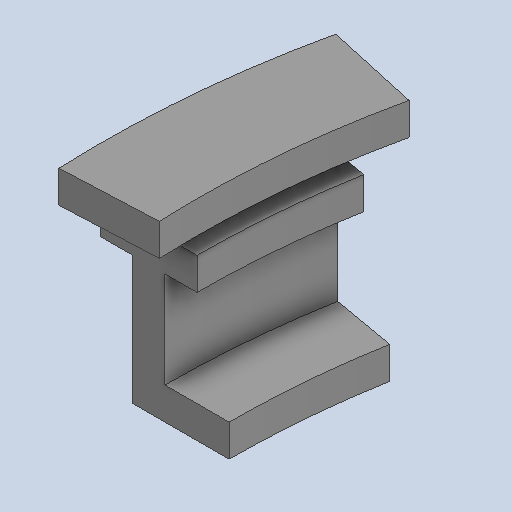
# Autodesk Inventor part: Moving Caoursel base Clip
Saved by Autodesk Inventor 2023 (Build 270158000, 158)
## iProperties
Created: 2023-02-14
Part Number: Moving Caoursel base Clip
Material: PLA Plastic
Document SubType Name: Modeling
Designer: cheng
Density: 1.25002 g/cm^3
Appearance: Generic
Author: cheng
Autodesk Inventor part; units mm, degrees
ref_plane "YZ Plane" through (0, 0, 0) normal (1, 0, 0) x (0, 1, 0)
ref_plane "XZ Plane" through (0, 0, 0) normal (0, 1, 0) x (-1, 0, 0)
ref_plane "XY Plane" through (0, 0, 0) normal (0, 0, 1) x (1, 0, 0)
sketch "Sketch1" plane through (0, 0, 0) normal (0, 1, 0) x (-1, 0, 0)
  circle A0 centre (0, 0) radius 285
  circle A1 centre (0, 0) radius 295
  circle A2 centre (0, 0) radius 275
  circle A3 centre (0, 0) radius 305
  line L0 (0, 0) -> (300.3664, -52.9627)
  line L1 (0, 0) -> (305, 0)
  point P0 (275, 0)
  point P1 (270.8221, -47.7532)
  dimension "d1" = 590
  dimension "d5" = 10
  dimension "d6" = 10
  dimension "d7" = 10
  dimension "d8" = 10
  constraints: 4 centre point, 4 coincident, 4 end point, 2 point on circle, 1 horizontal
  measures "d1" diameter of A1
  measures "d5" radial gap between concentric circles of A2 A0
  measures "d6" radial gap between concentric circles of A1 A0
  measures "d7" radial gap between concentric circles of A1 A3
  measures "d8" angle of L1 L0
extrude "Extrusion1" add sketch "Sketch1" along normal blind 10 contours L1 A1 L0 A0 | A0 L0 A2 L1 | L1 A3 L0 A1 picked at (291.5003, -5.7176) picked at (281.3509, -10.8537) picked at (297.9408, -46.5324)
sketch "Sketch2" plane through (0, 10, 0) normal (0, 1, 0) x (1, 0, 0)
  arc A0 (-270.8221, 47.7532) -> (-275, 0) centre (0, 0) ccw projected
  line L0 (-270.8221, 47.7532) -> (-300.3664, 52.9627) projected
  arc A1 (-300.3664, 52.9627) -> (-305, 0) centre (0, 0) ccw projected
  line L1 (-305, 0) -> (-275, 0) projected
  circle A2 centre (0, 0) radius 295
  circle A3 centre (0, 0) radius 285
  circle A4 centre (0, 0) radius 294.7
  circle A5 centre (0, 0) radius 285.3
  point P0 (-285, 0)
  point P1 (-280.6702, 49.4897)
  point P2 (-290.5183, 51.2262)
  point P3 (-295, 0)
  point P4 (-285.3, 0)
  point P5 (-280.9657, 49.5418)
  point P6 (-290.2228, 51.1741)
  point P7 (-294.7, 0)
  dimension "d11" = 10
  dimension "d12" = 590
  dimension "d26" = 0.3
  dimension "d27" = 0.3
  constraints: 4 centre point, 4 coincident
  measures "d11" radial gap between concentric circles of A3 A2
  measures "d12" diameter of A2
  measures "d26" radial gap between concentric circles of A3 A5
  measures "d27" radial gap between concentric circles of A2 A4
extrude "Extrusion2" add sketch "Sketch2" along normal blind 5.3 contours A5 L1 A4 L0 picked at (-291.2396, 11.2413)
sketch "Sketch3" plane through (0, 15.3, 0) normal (0, 1, 0) x (1, 0, 0)
  line L0 (-290.2228, 51.1741) -> (-300.3664, 52.9627) projected
  arc A0 (-300.3664, 52.9627) -> (-305, 0) centre (0, 0) ccw projected
  line L1 (-305, 0) -> (-294.7, 0) projected
  line L2 (-280.9657, 49.5418) -> (-290.2228, 51.1741) projected
  line L3 (-294.7, 0) -> (-285.3, 0) projected
  line L4 (-285.3, 0) -> (-275, 0) projected
  arc A1 (-270.8221, 47.7532) -> (-275, 0) centre (0, 0) ccw projected
  line L5 (-270.8221, 47.7532) -> (-280.9657, 49.5418) projected
  circle A2 centre (0, 0) radius 305
  circle A3 centre (0, 0) radius 275
  line L6 (0, 0) -> (-304.7097, -13.3039)
  line L7 (0, 0) -> (-297.7703, 66.0141)
  arc A4 (-300.3664, 52.9627) -> (-305, 0) centre (0, 0) ccw projected
  arc A5 (-270.8221, 47.7532) -> (-275, 0) centre (0, 0) ccw projected
  line L8 (-290.2228, 51.1741) -> (-300.3664, 52.9627) projected
  line L9 (-305, 0) -> (-294.7, 0) projected
  line L10 (-285.3, 0) -> (-275, 0) projected
  line L11 (-270.8221, 47.7532) -> (-280.9657, 49.5418) projected
  arc A6 (-290.2228, 51.1741) -> (-294.7, 0) centre (0, 0) ccw projected
  arc A7 (-280.9657, 49.5418) -> (-285.3, 0) centre (0, 0) ccw projected
  arc A8 (-290.2228, 51.1741) -> (-294.7, 0) centre (0, 0) ccw projected
  arc A9 (-280.9657, 49.5418) -> (-285.3, 0) centre (0, 0) ccw projected
  arc A10 (-290.2228, 51.1741) -> (-294.7, 0) centre (0, 0) ccw projected
  arc A11 (-280.9657, 49.5418) -> (-285.3, 0) centre (0, 0) ccw projected
  point P0 (-270.8221, 47.7532)
  point P1 (-268.4814, 59.5209)
  point P2 (-305, 0)
  point P3 (-274.7383, -11.9953)
  point P4 (-305, 0)
  point P5 (-300.3664, 52.9627)
  point P6 (-305, 0)
  point P7 (-270.8221, 47.7532)
  dimension "d23" = 2.5
  dimension "d28" = 2.5
  constraints: 4 end point, 3 point on circle, 2 centre point, 2 coincident, 1 concentric
  measures "d23" angle of L3 L6
  measures "d28" angle of L7 L5
extrude "Extrusion3" add sketch "Sketch3" along normal blind 10 contours A6 L1 A0 L0 | L0 A2 L7 A3 L5 L2 | L2 A7 L3 A6 | L5 A1 L4 A7 | L3 L4 A3 L6 A2 L1
sketch "Sketch4" plane through (0, 0, 0) normal (0, -1, 0) x (1, 0, 0)
  arc A0 (-275, 0) -> (-270.8221, -47.7532) centre (0, 0) ccw projected
  line L0 (-305, 0) -> (-275, 0) projected
  arc A1 (-305, 0) -> (-300.3664, -52.9627) centre (0, 0) ccw projected
  line L1 (-270.8221, -47.7532) -> (-300.3664, -52.9627) projected
  circle A2 centre (0, 0) radius 285
  circle A3 centre (0, 0) radius 295
  point P0 (-295, 0)
  point P1 (-290.5183, -51.2262)
  point P2 (-280.6702, -49.4897)
  point P3 (-285, 0)
  dimension "d17" = 10
  dimension "d18" = 590
  constraints: 2 centre point, 2 coincident
  measures "d17" radial gap between concentric circles of A3 A2
  measures "d18" diameter of A3
extrude "Extrusion4" add sketch "Sketch4" along normal blind 30 contours A2 L1 A3 L0 picked at (-291.3396, -11.2413)
sketch "Sketch5" plane through (0, -30, 0) normal (0, -1, 0) x (1, 0, 0)
  arc A0 (-295, 0) -> (-290.5183, -51.2262) centre (0, 0) ccw projected
  line L0 (-290.5183, -51.2262) -> (-280.6702, -49.4897) projected
  arc A1 (-285, 0) -> (-280.6702, -49.4897) centre (0, 0) ccw projected
  line L1 (-285, 0) -> (-295, 0) projected
  arc A2 (-295, 0) -> (-290.5183, -51.2262) centre (0, 0) ccw projected
  line L2 (-305, 0) -> (-295, 0) projected
  arc A3 (-305, 0) -> (-300.3664, -52.9627) centre (0, 0) ccw projected
  line L3 (-290.5183, -51.2262) -> (-300.3664, -52.9627) projected
  line L4 (-270.8221, -47.7532) -> (-280.6702, -49.4897) projected
  arc A4 (-275, 0) -> (-270.8221, -47.7532) centre (0, 0) ccw projected
  line L5 (-285, 0) -> (-275, 0) projected
  arc A5 (-305, 0) -> (-300.3664, -52.9627) centre (0, 0) ccw projected
  arc A6 (-275, 0) -> (-270.8221, -47.7532) centre (0, 0) ccw projected
  arc A7 (-285, 0) -> (-280.6702, -49.4897) centre (0, 0) ccw projected
  arc A8 (-295, 0) -> (-290.5183, -51.2262) centre (0, 0) ccw projected
  line L6 (-305, 0) -> (-295, 0) projected
  line L7 (-290.5183, -51.2262) -> (-300.3664, -52.9627) projected
  arc A9 (-285, 0) -> (-280.6702, -49.4897) centre (0, 0) ccw projected
  line L8 (-270.8221, -47.7532) -> (-280.6702, -49.4897) projected
  line L9 (-285, 0) -> (-275, 0) projected
  arc A10 (-295, 0) -> (-290.5183, -51.2262) centre (0, 0) ccw projected
  circle A11 centre (0, 0) radius 265
  line L10 (0, 0) -> (-305, 0)
  line L11 (0, 0) -> (-300.3664, -52.9627)
  point P0 (-290.5183, -51.2262)
  point P1 (-260.9741, -46.0168)
  point P2 (-265, 0)
  dimension "d25" = 30
  constraints: 4 end point, 1 centre point, 1 coincident, 1 horizontal
  measures "d25" radial gap between concentric circles of A0 A11
extrude "Extrusion5" add sketch "Sketch5" along normal blind 10 contours L1 A1 L0 A0 | L5 A4 L4 A1 | L10 A11 L11 A4
equation "\"d27\" = d26"
equation "\"d28\" = d23"
body "Solid1"
